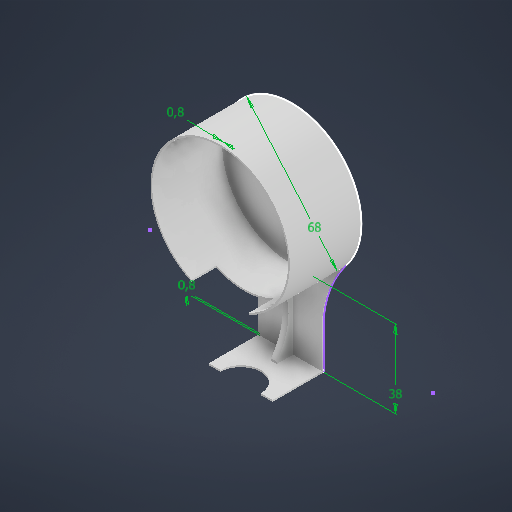
# Autodesk Inventor part: my_portafilter_holder
Saved by Autodesk Inventor 2026 (Build 300175000, 175)
## iProperties
Created: 2025-04-15
Part Number: my_portafilter_holder
Material: Generic
Document SubType Name: Modeling
Designer: Paul Juschitz
Density: 1 g/cm^3
Appearance: Default
Author: Paul Juschitz
Autodesk Inventor part; units mm, degrees
ref_plane "YZ Plane" through (0, 0, 0) normal (1, 0, 0) x (0, 1, 0)
ref_plane "XZ Plane" through (0, 0, 0) normal (0, 1, 0) x (-1, 0, 0)
ref_plane "XY Plane" through (0, 0, 0) normal (0, 0, 1) x (1, 0, 0)
sketch "Sketch1" plane through (0, 0, 0) normal (0, 0, 1) x (1, 0, 0)
  circle A0 centre (0, 0) radius 34
  line L0 (15.5526, -72) -> (-15.5526, -72)
  line L1 (-15.5526, -72) -> (-15.5526, -49.0211)
  line L2 (-15.5526, -26.0423) -> (15.5526, -72) construction
  line L3 (15.5526, -26.0423) -> (-15.5526, -72) construction
  line L4 (-10.1666, -34) -> (10.1666, -34)
  arc A1 (-15.5526, -49.0211) -> (-26.1483, -21.7317) centre (-69.1292, -54.1216) ccw
  arc A2 (26.1483, -21.7317) -> (15.5526, -49.0211) centre (69.1292, -54.1216) ccw
  line L5 (15.5526, -49.0211) -> (15.5526, -72)
  circle A3 centre (0, 0) radius 33.2
  line L6 (-15.5526, -71.2) -> (15.5526, -71.2)
  point P0 (0, -49.0211)
  point P1 (26.1483, -21.7317)
  dimension "d0" = 68
  dimension "d1" = 38
  dimension "d2" = 0.8
  dimension "d3" = 0.8
  constraints: 14 end point, 4 point on circle, 4 point on line, 3 centre point, 2 coincident, 2 horizontal, 2 midpoint, 1 parallel, 1 perpendicular, 3 other
  measures "d1" distance between parallel lines of L0 L4
  measures "d3" distance between parallel lines of L0 L6
extrude "Extrusion1" add sketch "Sketch1" along normal blind 0.8 contours A0 A2 L5 L6 L1 A1 | A3
extrude "Extrusion2" add sketch "Sketch1" along normal blind 25 contours L6 L5 L0 L1
extrude "Extrusion3" add sketch "Sketch1" along normal blind 35 contours A0
sketch "Sketch2" plane through (-15.5526, -72, 0) normal (0, -1, 0) x (1, 0, 0)
  line L0 (31.1053, 25) -> (0, 25) projected
  arc A0 (5.7113, 25) -> (25.3939, 25) centre (15.5526, 25) ccw
  line L1 (5.7113, 25) -> (25.3939, 25)
  point P0 (15.5526, 0)
  constraints: 2 end point, 2 point on circle, 2 point on line, 1 centre point, 1 midpoint
extrude "Extrusion4" cut sketch "Sketch2" against normal blind 2
sketch "Sketch3" plane through (0, 0, 0.8) normal (0, 0, 1) x (1, 0, 0)
  line L0 (-9.8413, -71.2) -> (9.8413, -71.2) projected
  line L1 (-1.3972, -33.6906) -> (1.3972, -33.6906)
  line L2 (1.3972, -33.6906) -> (1.3972, -71.2)
  line L3 (1.3972, -71.2) -> (-1.3972, -71.2)
  line L4 (-1.3972, -71.2) -> (-1.3972, -33.6906)
  line L5 (-1.3972, -33.6906) -> (1.3972, -71.2) construction
  line L6 (1.3972, -33.6906) -> (-1.3972, -71.2) construction
  point P0 (0, 0)
  point P1 (0, -52.4453)
  constraints: 12 end point, 2 midpoint, 2 parallel, 1 horizontal, 1 perpendicular, 1 point on line
extrude "Extrusion5" add sketch "Sketch3" along normal blind 8
sketch "Sketch4" plane through (1.3972, -71.2, 0.8) normal (1, 0, 0) x (0, 0, -1)
  point P0 (0.8, 71.2)
sketch "Sketch5" plane through (1.3972, -71.2, 0.8) normal (1, 0, 0) x (0, 0, -1)
  line L0 (-12.1, 0) -> (-14.4584, 0)
  arc A0 (-8.7861, 0) -> (-8.7861, 37.2287) centre (-31.8736, 18.6144) ccw
  line L1 (-8.7861, 37.374) -> (-8.7861, 37.374)
  line L2 (-8, 37.2287) -> (0, 37.2287) projected
  line L3 (-8.7861, 37.374) -> (-8.7861, 0)
  point P0 (0.8, 71.2)
  point P1 (-25, 0)
  point P2 (-24.2, 37.2287)
  constraints: 6 end point, 2 point on circle, 2 point on line, 1 centre point, 1 horizontal, 1 parallel, 1 perpendicular
extrude "Extrusion6" cut sketch "Sketch5" against normal up to surface (2.7945 mm away)
sketch "Sketch7" plane through (0, 0, 35) normal (0, 0, 1) x (1, 0, 0)
  line L0 (-14, -28.6906) -> (14, -28.6906)
  line L1 (14, -28.6906) -> (14, -38.6906)
  line L2 (14, -38.6906) -> (-14, -38.6906)
  line L3 (-14, -38.6906) -> (-14, -28.6906)
  line L4 (-1.3972, -33.6906) -> (1.3972, -33.6906) projected
  line L5 (-14, -28.6906) -> (14, -38.6906) construction
  line L6 (14, -28.6906) -> (-14, -38.6906) construction
  point P0 (0, 0)
  point P1 (0, -33.6906)
  dimension "d23" = 28
  dimension "d24" = 10
  constraints: 12 end point, 3 midpoint, 2 parallel, 1 horizontal, 1 perpendicular
  measures "d23" distance of L1.end L2.end
  measures "d24" distance of L0.end L1.end
extrude "Extrusion8" cut sketch "Sketch7" against normal blind 12
body "Solid1"
